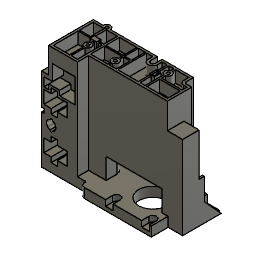
rightStepperBracket (Autodesk Fusion 360 design; units mm, degrees)
Autodesk Fusion 360 part; units mm, degrees
(part 1 of 3)
sketch "Sketch1" plane through (0, 0, 0) normal (0, 0, 1) x (1, 0, 0)
  line L0 (0, 0) -> (111.4, 0)
  line L1 (111.4, 0) -> (111.4, 93.5)
  line L2 (111.4, 93.5) -> (0, 93.5)
  line L3 (0, 93.5) -> (0, 0)
  line L4 (0, 71.5) -> (6, 71.5)
  line L5 (6, 71.5) -> (6, 93.5)
  line L6 (6, 93.5) -> (0, 93.5)
  line L7 (0, 93.5) -> (0, 71.5)
  line L8 (98.4, 93.5) -> (111.4, 93.5)
  line L9 (111.4, 93.5) -> (111.4, 71.5)
  line L10 (111.4, 71.5) -> (98.4, 71.5)
  line L11 (98.4, 71.5) -> (98.4, 93.5)
  line L12 (45.8, 8.3) -> (93.7, 8.3)
  line L13 (93.7, 8.3) -> (93.7, 26.1)
  line L14 (93.7, 26.1) -> (45.8, 26.1)
  line L15 (45.8, 26.1) -> (45.8, 8.3)
  line L16 (1.95, 58.65) -> (21.95, 58.65)
  line L17 (21.95, 58.65) -> (21.95, 47.65)
  line L18 (21.95, 47.65) -> (1.95, 47.65)
  line L19 (1.95, 47.65) -> (1.95, 58.65)
  line L20 (1.95, 22.7) -> (21.95, 22.7)
  line L21 (21.95, 22.7) -> (21.95, 11.7)
  line L22 (21.95, 11.7) -> (1.95, 11.7)
  line L23 (1.95, 11.7) -> (1.95, 22.7)
  point P0 (45.8, 17.2)
  point P1 (21.95, 17.2)
  dimension "d1" = 111.4
  dimension "d2" = 93.5
  dimension "d3" = 22
  dimension "d4" = 13
  dimension "d5" = 22
  dimension "d6" = 6
  dimension "d7" = 20
  dimension "d8" = 11
  dimension "d9" = 1.95
  dimension "d10" = 12.85
  dimension "d11" = 24.95
  dimension "d12" = 17.7
  dimension "d13" = 8.3
  dimension "d15" = 17.8
  dimension "d16" = 47.9
  constraint horizontal L0
  constraint vertical L1
  constraint horizontal L2
  constraint vertical L3
  constraint coincident L0.start L3.end
  constraint horizontal L4
  constraint vertical L5
  constraint horizontal L6
  constraint vertical L7
  constraint coincident L2 L5.end
  constraint coincident L3 L4.start
  constraint horizontal L8
  constraint vertical L9
  constraint horizontal L10
  constraint vertical L11
  constraint coincident L1 L9.end
  constraint coincident L2 L8.start
  constraint horizontal L12
  constraint vertical L13
  constraint horizontal L14
  constraint vertical L15
  constraint horizontal L16
  constraint vertical L17
  constraint horizontal L18
  constraint vertical L19
  constraint horizontal L20
  constraint vertical L21
  constraint horizontal L22
  constraint vertical L23
  constraint vertical L16.start L20.start
  constraint equal L16 L20
  constraint equal L17 L21
  constraint midpoint L15 P0
  constraint midpoint L21 P1
  constraint horizontal P0 P1
  measures "d1" distance of L0.start L0.end
  measures "d2" distance of L0.start L2.end
  measures "d3" distance of L8.start L10.end
  measures "d4" distance of L9.end L10.end
  measures "d5" distance of L4.end L5.end
  measures "d6" distance of L4.start L4.end
  measures "d7" distance of L16.start L16.end
  measures "d8" distance of L16.end L17.end
  measures "d9" distance of L3 L19
  measures "d10" distance of L4 L16
  measures "d11" distance of L18 L20
  measures "d12" distance of L1 L13
  measures "d13" distance of L0 L12
  measures "d15" distance of L12 L14
  measures "d16" distance of L13 L15
extrude "Extrude1" add sketch "Sketch1" along normal blind 42.8 contours L0 L1 L2 L3 L4 L5 L10 L11
sketch "Sketch2" plane through (0, 0, 42.8) normal (0, 0, 1) x (1, 0, 0)
  line L0 (21.95, 47.65) -> (1.95, 47.65)
  line L1 (1.95, 47.65) -> (1.95, 58.65)
  line L2 (1.95, 58.65) -> (21.95, 58.65)
  line L3 (21.95, 58.65) -> (21.95, 47.65)
  line L4 (45.8, 8.3) -> (45.8, 26.1)
  line L5 (45.8, 26.1) -> (93.7, 26.1)
  line L6 (93.7, 26.1) -> (93.7, 8.3)
  line L7 (93.7, 8.3) -> (45.8, 8.3)
  line L8 (21.95, 11.7) -> (1.95, 11.7)
  line L9 (1.95, 11.7) -> (1.95, 22.7)
  line L10 (1.95, 22.7) -> (21.95, 22.7)
  line L11 (21.95, 22.7) -> (21.95, 11.7)
  line L12 (0, 71.5) -> (0, 0)
  line L13 (0, 0) -> (111.4, 0)
  line L14 (111.4, 0) -> (111.4, 71.5)
  line L15 (111.4, 71.5) -> (98.4, 71.5)
  line L16 (98.4, 71.5) -> (98.4, 93.5)
  line L17 (98.4, 93.5) -> (6, 93.5)
  line L18 (6, 93.5) -> (6, 71.5)
  line L19 (6, 71.5) -> (0, 71.5)
  line L20 (30.75, 93.5) -> (111.4, 93.5)
  line L21 (111.4, 93.5) -> (111.4, 8.3)
  line L22 (111.4, 8.3) -> (30.75, 8.3)
  line L23 (30.75, 8.3) -> (30.75, 93.5)
  line L24 (38.2, 8.3) -> (99, 8.3)
  line L25 (99, 8.3) -> (99, 0)
  line L26 (99, 0) -> (38.2, 0)
  line L27 (38.2, 0) -> (38.2, 8.3)
  dimension "d19" = 30.75
  dimension "d23" = 12.4
  dimension "d24" = 60.8
  constraint horizontal L20
  constraint vertical L21
  constraint horizontal L22
  constraint vertical L23
  constraint coincident L14 L21.end
  constraint coincident L17 L20.start
  constraint collinear L7 L22
  constraint horizontal L24
  constraint vertical L25
  constraint horizontal L26
  constraint vertical L27
  constraint coincident L13 L25.end
  constraint coincident L22 L24.start
  measures "d19" distance of L12 L23
  measures "d23" distance of L14 L25
  measures "d24" distance of L25.end L26.end
extrude "Extrude2" cut sketch "Sketch2" against normal blind 9.5 contours L4 L5 L6 L14 L15 L16 L17 L20 L21 L22 L23 L24 | L13 L14 L22 L25
extrude "Extrude3" add sketch "Sketch2" along normal blind 5 contours L7 L13 L22 L24 L25 L26 L27
sketch "Sketch3" plane through (0, 0, 42.8) normal (0, 0, 1) x (1, 0, 0)
  line L0 (38.2, 0) -> (38.2, 8.3)
  line L1 (38.2, 8.3) -> (30.75, 8.3)
  line L2 (30.75, 8.3) -> (30.75, 93.5)
  line L3 (30.75, 93.5) -> (6, 93.5)
  line L4 (6, 93.5) -> (6, 71.5)
  line L5 (6, 71.5) -> (0, 71.5)
  line L6 (0, 71.5) -> (0, 0)
  line L7 (0, 0) -> (38.2, 0)
  line L8 (21.95, 47.65) -> (1.95, 47.65)
  line L9 (1.95, 47.65) -> (1.95, 58.65)
  line L10 (1.95, 58.65) -> (21.95, 58.65)
  line L11 (21.95, 58.65) -> (21.95, 47.65)
  line L12 (21.95, 11.7) -> (1.95, 11.7)
  line L13 (1.95, 11.7) -> (1.95, 22.7)
  line L14 (1.95, 22.7) -> (21.95, 22.7)
  line L15 (21.95, 22.7) -> (21.95, 11.7)
  line L16 (8.2, 58.65) -> (13.55, 58.65)
  line L17 (13.55, 58.65) -> (13.55, 62.9)
  line L18 (13.55, 62.9) -> (8.2, 62.9)
  line L19 (8.2, 62.9) -> (8.2, 58.65)
  line L20 (8.2, 47.65) -> (13.55, 47.65)
  line L21 (13.55, 47.65) -> (13.55, 43.4)
  line L22 (13.55, 43.4) -> (8.2, 43.4)
  line L23 (8.2, 43.4) -> (8.2, 47.65)
  line L24 (8.2, 22.7) -> (13.55, 22.7)
  line L25 (13.55, 22.7) -> (13.55, 26.95)
  line L26 (13.55, 26.95) -> (8.2, 26.95)
  line L27 (8.2, 26.95) -> (8.2, 22.7)
  line L28 (8.2, 11.7) -> (13.55, 11.7)
  line L29 (13.55, 11.7) -> (13.55, 7.45)
  line L30 (13.55, 7.45) -> (8.2, 7.45)
  line L31 (8.2, 7.45) -> (8.2, 11.7)
  circle A0 centre (8.25, 35.175) radius 4
  line L32 (21.95, 47.65) -> (21.95, 22.7) construction
  line L33 (9.3, 68.2) -> (2, 68.2)
  line L34 (2, 68.2) -> (2, 60.65)
  line L35 (2, 60.65) -> (6.2, 60.65)
  line L36 (6.2, 60.65) -> (6.2, 64.9)
  line L37 (6.2, 64.9) -> (15.55, 64.9)
  line L38 (28.75, 81.5) -> (9.3, 81.5)
  line L39 (9.3, 81.5) -> (9.3, 68.2)
  line L40 (28.75, 81.5) -> (28.75, 60.65)
  line L41 (28.75, 60.65) -> (15.55, 60.65)
  line L42 (15.55, 60.65) -> (15.55, 64.9)
  circle A1 centre (8.25, 31.175) radius 1
  circle A2 centre (8.25, 39.175) radius 1
  circle A3 centre (8.25, 35.175) radius 1.5
  line L43 (6.125, 39.175) -> (10.375, 39.175)
  line L44 (10.375, 39.175) -> (10.375, 31.175)
  line L45 (10.375, 31.175) -> (6.125, 31.175)
  line L46 (6.125, 31.175) -> (6.125, 39.175)
  point P0 (11.95, 7.2)
  point P1 (11.95, 11.45)
  point P2 (11.95, 26.7)
  point P3 (11.95, 22.45)
  point P4 (11.95, 62.9)
  point P5 (11.95, 58.65)
  point P6 (11.95, 43.4)
  point P7 (11.95, 47.65)
  point P8 (21.95, 35.175)
  point P9 (8.25, 39.175)
  point P10 (8.25, 31.175)
  dimension "d27" = 5.35
  dimension "d28" = 19.5
  dimension "d29" = 8.2
  dimension "d30" = 8
  dimension "d31" = 8.25
  dimension "d32" = 12
  dimension "d33" = 2
  dimension "d34" = 2
  dimension "d35" = 2
  dimension "d36" = 2
  dimension "d37" = 2
  dimension "d38" = 2
  dimension "d39" = 2
  dimension "d40" = 3.3
  dimension "d41" = 3.3
  dimension "d47" = 2
  dimension "d48" = 2
  dimension "d49" = 3
  dimension "d50" = 4.25
  constraint horizontal L16
  constraint vertical L17
  constraint horizontal L18
  constraint vertical L19
  constraint coincident L10 L16.start
  constraint horizontal L20
  constraint vertical L21
  constraint horizontal L22
  constraint vertical L23
  constraint coincident L8 L20.start
  constraint horizontal L24
  constraint vertical L25
  constraint horizontal L26
  constraint vertical L27
  constraint coincident L14 L24.start
  constraint horizontal L28
  constraint vertical L29
  constraint horizontal L30
  constraint vertical L31
  constraint coincident L12 L28.start
  constraint vertical P0 P1
  constraint vertical P2 P3
  constraint vertical P4 P5
  constraint vertical P6 P7
  constraint equal L18 L22
  constraint equal L17 L21
  constraint equal L21 L25
  constraint equal L25 L29
  constraint equal L24 L30
  constraint equal L18 L26
  constraint vertical L24.start L28.start
  constraint vertical L22.end L26.end
  constraint vertical L16.start L20.start
  constraint coincident L8.start L11.end
  constraint coincident L14.end L15.start
  constraint midpoint L32 P8
  constraint horizontal A0.centre P8
  constraint horizontal L33
  constraint perpendicular L33 L34
  constraint perpendicular L34 L35
  constraint perpendicular L33 L36
  constraint perpendicular L36 L37
  constraint perpendicular L33 L39
  constraint perpendicular L37 L40
  constraint perpendicular L17 L41
  constraint perpendicular L37 L42
  constraint coincident L38.start L40.start
  constraint coincident A0 P10
  constraint coincident A0 P9
  constraint vertical A0.centre P9
  constraint vertical A0.centre P10
  constraint concentric A0 A3
  constraint horizontal L43
  constraint vertical L44
  constraint horizontal L45
  constraint vertical L46
  constraint midpoint L43 P9
  constraint coincident P9 A2.centre
  constraint midpoint L45 P10
  constraint coincident P10 A1.centre
  measures "d27" distance of L17.end L18.end
  measures "d28" distance of L18 L22
  measures "d29" distance of L6 L27
  measures "d30" diameter of A0
  measures "d31" distance of L6 A0.centre
  measures "d32" distance of L3 L38
  measures "d33" distance of L6 L34
  measures "d34" distance of L10 L35
  measures "d35" distance of L19 L36
  measures "d36" distance of L18 L37
  measures "d37" distance of L17 L42
  measures "d38" distance of L10 L41
  measures "d39" distance of L2 L40
  measures "d40" distance of L5 L33
  measures "d41" distance of L4 L39
  measures "d47" diameter of A1
  measures "d48" diameter of A2
  measures "d49" diameter of A3
  measures "d50" distance of L44 L46
extrude "Extrude4" cut sketch "Sketch3" against normal blind 29 contours L8 L20 L21 L22 L23 | L10 L16 L17 L18 L19 | L12 L28 L29 L30 L31 | L14 L24 L25 L26 L27
extrude "Extrude5" cut sketch "Sketch3" against normal blind 9.6 contours L33 L34 L35 L36 L37 L38 L39 L40 L41 L42
extrude "Extrude6" cut sketch "Sketch3" against normal blind 25 contours A0 A1 A2 L44 L46 | A0 A2 | A0 A2 L43 | A0 A1 L45 | A0 A1 | A0 A2 L43 | A2 L43 | A0 A1 L45 | A1 L45 | A3
extrude "Extrude7" cut sketch "Sketch3" against normal up to surface (42.8 mm away) contours A3
extrude "Extrude8" cut sketch "Sketch3" against normal blind 15.15 contours A0 L44 | A0 L46
sketch "Sketch4" plane through (0, 0, 0) normal (0, 0, -1) x (-1, 0, 0)
  circle A0 centre (-8.25, 35.175) radius 1.5
  line L0 (-1.95, 47.65) -> (-21.95, 47.65)
  line L1 (-21.95, 47.65) -> (-21.95, 58.65)
  line L2 (-21.95, 58.65) -> (-1.95, 58.65)
  line L3 (-1.95, 58.65) -> (-1.95, 47.65)
  line L4 (-45.8, 26.1) -> (-45.8, 8.3)
  line L5 (-45.8, 8.3) -> (-93.7, 8.3)
  line L6 (-93.7, 8.3) -> (-93.7, 26.1)
  line L7 (-93.7, 26.1) -> (-45.8, 26.1)
  line L8 (-1.95, 11.7) -> (-21.95, 11.7)
  line L9 (-21.95, 11.7) -> (-21.95, 22.7)
  line L10 (-21.95, 22.7) -> (-1.95, 22.7)
  line L11 (-1.95, 22.7) -> (-1.95, 11.7)
  line L12 (0, 0) -> (0, 71.5)
  line L13 (0, 71.5) -> (-6, 71.5)
  line L14 (-6, 71.5) -> (-6, 93.5)
  line L15 (-6, 93.5) -> (-98.4, 93.5)
  line L16 (-98.4, 93.5) -> (-98.4, 71.5)
  line L17 (-98.4, 71.5) -> (-111.4, 71.5)
  line L18 (-111.4, 71.5) -> (-111.4, 0)
  line L19 (-111.4, 0) -> (0, 0)
  line L20 (-97.3, 1.8) -> (-40.3, 1.8)
  line L21 (-40.3, 1.8) -> (-40.3, 32.85)
  line L22 (-97.3, 32.85) -> (-97.3, 1.8)
  circle A1 centre (-68.565, 5.235) radius 1.2
  circle A2 centre (-57.165, 5.235) radius 1.2
  line L23 (-97.3, 32.85) -> (-40.3, 32.85)
  circle A3 centre (-68.565, 29.235) radius 1.2
  circle A4 centre (-57.165, 29.235) radius 1.2
  circle A5 centre (-68.565, 29.235) radius 3.3
  circle A6 centre (-57.165, 29.235) radius 3.3
  circle A7 centre (-68.565, 5.235) radius 3.3
  circle A8 centre (-57.165, 5.235) radius 3.3
  dimension "d57" = 14.1
  dimension "d58" = 57
  dimension "d59" = 1.8
  dimension "d60" = 11.4
  dimension "d61" = 28.735
  dimension "d63" = 3.065
  dimension "d64" = 2.4
  dimension "d65" = 6.75
  dimension "d67" = 6.6
  dimension "d68" = 24
  constraint horizontal L20
  constraint vertical L21
  constraint vertical L22
  constraint equal A1 A2
  constraint horizontal A1.centre A2.centre
  constraint perpendicular L22 L23
  constraint vertical A1.centre A3.centre
  constraint vertical A2.centre A4.centre
  constraint horizontal A3.centre A4.centre
  constraint equal A3 A4
  constraint equal A1 A3
  constraint concentric A3 A5
  constraint concentric A4 A6
  constraint equal A5 A6
  constraint concentric A1 A7
  constraint concentric A2 A8
  constraint equal A6 A8
  constraint equal A7 A8
  measures "d57" distance of L18 L22
  measures "d58" distance of L21 L22
  measures "d59" distance of L19 L20
  measures "d60" distance of A1.centre A2.centre
  measures "d61" distance of L22 A1.centre
  measures "d63" distance of L5 A1.centre
  measures "d64" diameter of A1
  measures "d65" distance of L7 L23
  measures "d67" diameter of A5
  measures "d68" distance of A1.centre A3.centre
extrude "Extrude9" cut sketch "Sketch4" against normal blind 2 contours L7 A6 | L5 A8 | L7 A5 | L5 A7 | L20 L21 L22 L23 | A1 | A2 | A3 | A4 picked at (-57.1351, 26.7461) picked at (-57.1949, 7.6772) picked at (-68.5949, 26.7461) picked at (-68.5949, 7.6772)
extrude "Extrude10" cut sketch "Sketch4" against normal blind 9 from surface at -2 contours A1 | A2 | A3 | A4
sketch "Sketch6" plane through (0, 0, 0) normal (0, 0, -1) x (-1, 0, 0)
  line L0 (-40.3, 32.85) -> (-40.3, 1.8)
  line L1 (-40.3, 1.8) -> (-97.3, 1.8)
  line L2 (-97.3, 1.8) -> (-97.3, 32.85)
  line L3 (-97.3, 32.85) -> (-40.3, 32.85)
  circle A0 centre (-8.25, 35.175) radius 1.5
  line L4 (-1.95, 47.65) -> (-21.95, 47.65)
  line L5 (-21.95, 47.65) -> (-21.95, 58.65)
  line L6 (-21.95, 58.65) -> (-1.95, 58.65)
  line L7 (-1.95, 58.65) -> (-1.95, 47.65)
  line L8 (-1.95, 11.7) -> (-21.95, 11.7)
  line L9 (-21.95, 11.7) -> (-21.95, 22.7)
  line L10 (-21.95, 22.7) -> (-1.95, 22.7)
  line L11 (-1.95, 22.7) -> (-1.95, 11.7)
  line L12 (0, 0) -> (0, 71.5)
  line L13 (0, 71.5) -> (-6, 71.5)
  line L14 (-6, 71.5) -> (-6, 93.5)
  line L15 (-6, 93.5) -> (-98.4, 93.5)
  line L16 (-98.4, 93.5) -> (-98.4, 71.5)
  line L17 (-98.4, 71.5) -> (-111.4, 71.5)
  line L18 (-111.4, 71.5) -> (-111.4, 0)
  line L19 (-111.4, 0) -> (0, 0)
  line L20 (-98.4, 71.5) -> (-98.4, 26.1)
  line L21 (-98.4, 26.1) -> (-93.7, 26.1)
  line L22 (-93.7, 26.1) -> (-93.7, 8.3)
  line L23 (-93.7, 8.3) -> (-99.3, 8.3)
  line L24 (-99.3, 8.3) -> (-99.3, 1.6)
  line L25 (-99.3, 1.6) -> (-109.65, 1.6)
  line L26 (-109.65, 1.6) -> (-109.65, 34.9)
  line L27 (-109.65, 34.9) -> (-111.4, 34.9)
  point P0 (-93.7, 8.3)
  point P1 (-93.7, 26.1)
  dimension "d80" = 34.9
  dimension "d81" = 1.75
  dimension "d82" = 1.6
  dimension "d83" = 2
  constraint coincident L16.end L17.start
  constraint perpendicular L17 L20
  constraint coincident P1 L21.end
  constraint perpendicular L2 L21
  constraint coincident P0 L22.end
  constraint perpendicular L2 L23
  constraint perpendicular L23 L24
  constraint perpendicular L2 L25
  constraint perpendicular L25 L26
  constraint coincident L18 L27.end
  constraint perpendicular L18 L27
  measures "d80" distance of L18.end L27.end
  measures "d81" distance of L18 L26
  measures "d82" distance of L19 L25
  measures "d83" distance of L2 L24
extrude "Extrude11" cut sketch "Sketch6" against normal blind 19.1 contours L2 L21 L22 L23 | L2 L17 L18 L20 L21 L23 L24 L25 L26 L27
sketch "Sketch5" plane through (0, 8.3, 0) normal (0, 1, 0) x (-1, 0, 0)
  line L0 (-97.3, 2) -> (-45.8, 2)
  line L1 (-45.8, 2) -> (-45.8, 33.3)
  line L2 (-45.8, 33.3) -> (-30.75, 33.3)
  line L3 (-30.75, 33.3) -> (-30.75, 42.8)
  line L4 (-30.75, 42.8) -> (-38.2, 42.8)
  line L5 (-38.2, 42.8) -> (-38.2, 47.8)
  line L6 (-38.2, 47.8) -> (-99, 47.8)
  line L7 (-99, 47.8) -> (-99, 33.3)
  line L8 (-99, 33.3) -> (-93.7, 33.3)
  line L9 (-93.7, 33.3) -> (-93.7, 19.1)
  circle A0 centre (-78.55, 26.05) radius 12
  circle A1 centre (-63.05, 41.55) radius 1.75
  circle A2 centre (-94.05, 41.55) radius 1.75
  circle A3 centre (-94.05, 10.55) radius 1.75
  circle A4 centre (-63.05, 10.55) radius 1.75
  line L10 (-63.05, 10.55) -> (-63.05, 41.55) construction
  line L11 (-63.05, 41.55) -> (-94.05, 41.55) construction
  line L12 (-111.4, 0) -> (-111.4, 33.3) construction
  line L13 (-93.7, 19.1) -> (-99.3, 19.1)
  line L14 (-99.3, 19.1) -> (-99.3, 0)
  line L15 (-99.3, 0) -> (-97.3, 0)
  line L16 (-97.3, 0) -> (-97.3, 2)
  circle A5 centre (-63.05, 41.55) radius 3.25
  circle A6 centre (-94.05, 41.55) radius 3.25
  circle A7 centre (-94.05, 10.55) radius 3.25
  circle A8 centre (-63.05, 10.55) radius 3.25
  line L17 (-59.8, 10.55) -> (-59.8, 2)
  line L18 (-66.3, 10.55) -> (-66.3, 2)
  line L19 (-59.8, 41.55) -> (-59.8, 47.8)
  line L20 (-66.3, 41.55) -> (-66.3, 47.8)
  line L21 (-90.8, 41.55) -> (-90.8, 47.8)
  line L22 (-97.3, 41.55) -> (-97.3, 47.8)
  line L23 (-97.3, 10.55) -> (-97.3, 0)
  line L24 (-90.8, 10.55) -> (-90.8, 2)
  point P0 (-63.05, 26.05)
  point P1 (-78.55, 41.55)
  dimension "d75" = 24
  dimension "d76" = 3.5
  dimension "d86" = 6.5
  dimension "d87" = 6.25
  dimension "d88" = 31
  constraint equal A3 A4
  constraint equal A1 A4
  constraint equal A1 A2
  constraint horizontal A3.centre A4.centre
  constraint vertical A2.centre A3.centre
  constraint horizontal A1.centre A2.centre
  constraint vertical A1.centre A4.centre
  constraint coincident A4.centre L10.start
  constraint coincident A1.centre L10.end
  constraint coincident A2.centre L11.end
  constraint midpoint L10 P0
  constraint horizontal A0.centre P0
  constraint midpoint L11 P1
  constraint vertical A0.centre P1
  constraint equal L10 L11
  constraint concentric A3 A7
  constraint equal A7 A8
  constraint equal A6 A7
  constraint equal A5 A6
  constraint coincident A8 L17.start
  constraint coincident L0 L17.end
  constraint tangent A8 L17
  constraint perpendicular L0 L17
  constraint coincident A8 L18.start
  constraint coincident L0 L18.end
  constraint tangent A8 L18
  constraint perpendicular L0 L18
  constraint coincident A5 L19.start
  constraint coincident L6 L19.end
  constraint tangent A5 L19
  constraint perpendicular L6 L19
  constraint coincident A5 L20.start
  constraint coincident L11 L20.start
  constraint coincident L6 L20.end
  constraint tangent A5 L20
  constraint coincident L11 L21.start
  constraint coincident A6 L21.start
  constraint coincident L6 L21.end
  constraint tangent A6 L21
  constraint coincident A6 L22.start
  constraint coincident L6 L22.end
  constraint tangent A6 L22
  constraint perpendicular L6 L22
  constraint coincident A7 L23.start
  constraint coincident L15.end L16.start
  constraint perpendicular L0 L23
  constraint coincident A7 L24.start
  constraint coincident L0 L24.end
  constraint tangent A7 L24
  constraint perpendicular L0 L24
  measures "d75" diameter of A0
  measures "d76" diameter of A4
  measures "d86" diameter of A5
  measures "d87" distance of L19.start L19.end
  measures "d88" distance of A1.centre A2.centre
extrude "Extrude12" cut sketch "Sketch5" against normal up to surface (8.3 mm away) contours A0 | A1 | A2 | A3 | A4
extrude "Extrude13" cut sketch "Sketch5" against normal blind 4.9 contours L0 A7 L23 L24 | A7 | L0 A8 L17 L18 | A8 | L6 A6 L21 L22 | A6 | L6 A5 L19 L20 | A5
sketch "Sketch7" plane through (0, 58.65, 0) normal (0, -1, 0) x (1, 0, 0)
  line L0 (8.2, 13.8) -> (8.2, 42.8)
  line L1 (8.2, 42.8) -> (1.95, 42.8)
  line L2 (1.95, 42.8) -> (1.95, 0)
  line L3 (1.95, 0) -> (21.95, 0)
  line L4 (21.95, 0) -> (21.95, 42.8)
  line L5 (21.95, 42.8) -> (13.55, 42.8)
  line L6 (13.55, 42.8) -> (13.55, 13.8)
  line L7 (13.55, 13.8) -> (8.2, 13.8)
  circle A0 centre (10.875, 8.975) radius 2.525
  line L8 (13.4, 8.975) -> (13.4, 0)
  line L9 (8.35, 8.975) -> (8.35, 0)
  circle A1 centre (10.875, 10.3) radius 3.5
  line L10 (13.55, 13.8) -> (13.55, 12.5571)
  line L11 (8.2, 13.8) -> (8.2, 12.5571)
  line L12 (11.625, 11.5) -> (10.125, 11.5)
  line L13 (10.125, 11.5) -> (10.125, 5)
  line L14 (10.125, 5) -> (11.625, 5)
  line L15 (11.625, 5) -> (11.625, 11.5)
  line L16 (8.35, 0) -> (13.4, 0) construction
  line L17 (13.4, 0) -> (8.35, 0) construction
  point P0 (10.875, 5)
  point P1 (10.875, 0)
  point P2 (10.875, 13.8)
  dimension "d93" = 5.05
  dimension "d94" = 8.975
  dimension "d95" = 7
  dimension "d96" = 1.5
  dimension "d97" = 6.5
  constraint coincident A0 L8.start
  constraint coincident L3 L8.end
  constraint tangent A0 L8
  constraint perpendicular L3 L8
  constraint coincident A0 L9.start
  constraint coincident L3 L9.end
  constraint tangent A0 L9
  constraint perpendicular L3 L9
  constraint tangent L7 A1
  constraint coincident L6.end L7.start
  constraint coincident A1 L10.end
  constraint perpendicular L7 L10
  constraint coincident L0.start L7.end
  constraint coincident A1 L11.end
  constraint perpendicular L7 L11
  constraint horizontal L12
  constraint vertical L13
  constraint horizontal L14
  constraint vertical L15
  constraint tangent A0 L12
  constraint midpoint L14 P0
  constraint vertical A0.centre P0
  constraint midpoint L17 P1
  constraint midpoint L7 P2
  constraint vertical P1 P2
  constraint vertical A1.centre P1
  measures "d93" diameter of A0
  measures "d94" distance of L8.start L8.end
  measures "d95" diameter of A1
  measures "d96" distance of L13.end L14.end
  measures "d97" distance of L12.end L13.end
extrude "Extrude14" cut sketch "Sketch7" against normal blind 4 contours L7 A1 L11 | L7 A1 L10 | L3 A0 L8 L9 A1 L13 L14 L15 | A0 L9 A1 | A0 A1 L13 | A0 A1 L13 | A0 L8 A1 | A0 A1 L13 L15 | A0 A1 L13 L15 | A0 L13 L14 L15 | A0 A1 L15 | A0 A1 L15
extrude "Extrude15" cut 2 faces at (13.1796, 62.65, 13.3159) (8.5704, 62.65, 13.3159) along direction (0, -1, 0) up to surface end surface through (13.55, 62.9, 42.8) normal (0, -1, 0) offset 0
extrude "Extrude16" add sketch "Sketch7" along normal blind 0.95 from surface at -4 contours A0 A1 L13 L15 | A0 A1 L13 L15 | A0 L13 L14 L15
chamfer "Chamfer1" distance 0.95 angle 45 1 edges at (10.875, 61.7, 5)
sketch "Sketch8" plane through (0, 22.7, 0) normal (0, -1, 0) x (1, 0, 0)
  line L0 (8.2, 13.8) -> (8.2, 42.8)
  line L1 (8.2, 42.8) -> (1.95, 42.8)
  line L2 (1.95, 42.8) -> (1.95, 0)
  line L3 (1.95, 0) -> (21.95, 0)
  line L4 (21.95, 0) -> (21.95, 42.8)
  line L5 (21.95, 42.8) -> (13.55, 42.8)
  line L6 (13.55, 42.8) -> (13.55, 13.8)
  line L7 (13.55, 13.8) -> (8.2, 13.8)
  line L8 (11.625, 5) -> (11.625, 11.5)
  line L9 (11.625, 11.5) -> (10.125, 11.5)
  line L10 (8.2, 13.8) -> (8.2, 12.5571)
  line L11 (10.125, 11.5) -> (10.125, 5)
  line L12 (13.55, 13.8) -> (13.55, 12.5571)
  circle A0 centre (10.875, 8.975) radius 2.525
  line L13 (13.55, 13.8) -> (8.2, 13.8)
  line L14 (13.4, 8.975) -> (13.4, 0)
  circle A1 centre (10.875, 10.3) radius 3.5
  line L15 (8.35, 8.975) -> (8.35, 0)
  line L16 (10.125, 5) -> (11.625, 5)
  line L17 (8.35, 0) -> (13.4, 0) construction
  point P0 (10.875, 5)
  point P1 (13.55, 13.8)
  point P2 (10.875, 0)
  point P3 (10.875, 13.8)
  dimension "d106" = 5.05
  dimension "d107" = 8.975
  dimension "d108" = 7
  dimension "d109" = 1.5
  dimension "d110" = 6.5
  constraint coincident L14.start A0
  constraint tangent A0 L14
  constraint coincident L15.start A0
  constraint tangent A0 L15
  constraint tangent L13 A1
  constraint coincident P1 L6.end
  constraint coincident L12.end A1
  constraint perpendicular L12 L13
  constraint coincident L0.start L7.end
  constraint coincident L10.end A1
  constraint perpendicular L10 L13
  constraint horizontal L9
  constraint vertical L11
  constraint horizontal L16
  constraint vertical L8
  constraint tangent L9 A0
  constraint midpoint P0 L16
  constraint vertical A0.centre P0
  constraint coincident L3 L14.end
  constraint coincident L3 L15.end
  constraint vertical A0.centre A1.centre
  constraint coincident L0 L7.end
  constraint collinear L0 L10
  constraint perpendicular L3 L14
  constraint perpendicular L3 L15
  constraint midpoint L17 P2
  constraint midpoint L7 P3
  constraint vertical P2 P3
  measures "d106" diameter of A0
  measures "d107" distance of L14.start L14.end
  measures "d108" diameter of A1
  measures "d109" distance of L11.end L8.start
  measures "d110" distance of L11.end L9.end
extrude "Extrude17" cut sketch "Sketch8" against normal blind 4 contours L7 L10 L13 A1 | L7 L12 L13 A1 | A0 A1 L15 | L3 L8 L11 A0 L14 A1 L15 L16 | L11 A0 A1 | L11 A0 A1 | A0 L14 A1 | L8 L11 A0 L16 | L8 L11 A0 A1 | L8 L11 A0 A1 | L8 A0 A1 | L8 A0 A1
extrude "Extrude18" cut 2 faces at (13.1796, 26.7, 13.3159) (8.5704, 26.7, 13.3159) along direction (0, -1, 0) up to surface end surface through (13.55, 26.95, 42.8) normal (0, -1, 0) offset 0
extrude "Extrude19" add sketch "Sketch8" along normal blind 0.95 from surface at -4 contours L8 L11 A0 L16 | L8 L11 A0 A1 | L8 L11 A0 A1
chamfer "Chamfer2" distance 0.95 angle 45 1 edges at (10.875, 25.75, 5)
sketch "Sketch9" plane through (0, 11.7, 0) normal (0, 1, 0) x (-1, 0, 0)
  line L0 (-8.2, 42.8) -> (-8.2, 13.8)
  line L1 (-8.2, 13.8) -> (-13.55, 13.8)
  line L2 (-13.55, 13.8) -> (-13.55, 42.8)
  line L3 (-13.55, 42.8) -> (-21.95, 42.8)
  line L4 (-21.95, 42.8) -> (-21.95, 0)
  line L5 (-21.95, 0) -> (-1.95, 0)
  line L6 (-1.95, 0) -> (-1.95, 42.8)
  line L7 (-1.95, 42.8) -> (-8.2, 42.8)
  line L8 (-13.55, 13.8) -> (-13.55, 12.5571)
  line L9 (-13.4, 8.975) -> (-13.4, 0)
  line L10 (-8.2, 13.8) -> (-13.55, 13.8)
  circle A0 centre (-10.875, 8.975) radius 2.525
  line L11 (-10.125, 5) -> (-10.125, 11.5)
  line L12 (-8.35, 8.975) -> (-8.35, 0)
  line L13 (-11.625, 5) -> (-10.125, 5)
  line L14 (-10.125, 11.5) -> (-11.625, 11.5)
  line L15 (-8.2, 13.8) -> (-8.2, 12.5571)
  line L16 (-11.625, 11.5) -> (-11.625, 5)
  line L17 (-13.4, 0) -> (-8.35, 0) construction
  circle A1 centre (-10.875, 10.3) radius 3.5
  point P0 (-10.875, 13.8)
  point P1 (-10.875, 0)
  point P2 (-8.2, 13.8)
  point P3 (-10.875, 5)
  point P4 (-10.875, 13.8)
  dimension "d119" = 5.05
  dimension "d120" = 8.975
  dimension "d121" = 7
  dimension "d122" = 1.5
  dimension "d123" = 6.5
  constraint coincident L12.start A0
  constraint tangent A0 L12
  constraint coincident L9.start A0
  constraint tangent L9 A0
  constraint tangent L10 A1
  constraint coincident P2 L0.end
  constraint coincident L15.end A1
  constraint perpendicular L10 L15
  constraint coincident L1.end L2.start
  constraint coincident L8.end A1
  constraint perpendicular L8 L10
  constraint horizontal L14
  constraint vertical L16
  constraint horizontal L13
  constraint vertical L11
  constraint tangent A0 L14
  constraint midpoint P3 L13
  constraint vertical P3 A0.centre
  constraint vertical A1.centre A0.centre
  constraint midpoint P1 L17
  constraint vertical P4 P1
  constraint perpendicular L12 L17
  constraint perpendicular L9 L17
  constraint collinear L5 L17
  constraint midpoint L1 P4
  constraint vertical P1 P4
  constraint coincident L0.end L1.start
  measures "d119" diameter of A0
  measures "d120" distance of L12.start L12.end
  measures "d121" diameter of A1
  measures "d122" distance of L13.start L11.start
  measures "d123" distance of L14.end L13.start
extrude "Extrude20" cut sketch "Sketch9" against normal blind 4 contours L1 L10 L15 A1 | L1 L8 L10 A1 | L5 L9 A0 L11 L12 L13 L16 A1 | L9 A0 A1 | A0 L12 A1 | A0 L16 A1 | A0 L16 A1 | A0 L11 A1 | A0 L11 A1 | A0 L11 L16 A1 | A0 L11 L16 A1 | A0 L11 L13 L16
extrude "Extrude21" cut 2 faces at (8.5704, 7.7, 13.3159) (13.1796, 7.7, 13.3159) along direction (0, 1, 0) up to surface end surface through (13.55, 7.45, 42.8) normal (0, 1, 0) offset 0
extrude "Extrude22" add sketch "Sketch9" along normal blind 0.95 from surface at -4 contours A0 L11 L16 A1 | A0 L11 L16 A1 | A0 L11 L13 L16
chamfer "Chamfer3" distance 0.95 angle 45 1 edges at (10.875, 8.65, 5)
sketch "Sketch10" plane through (0, 47.65, 0) normal (0, 1, 0) x (-1, 0, 0)
  line L0 (-8.2, 42.8) -> (-8.2, 13.8)
  line L1 (-8.2, 13.8) -> (-13.55, 13.8)
  line L2 (-13.55, 13.8) -> (-13.55, 42.8)
  line L3 (-13.55, 42.8) -> (-21.95, 42.8)
  line L4 (-21.95, 42.8) -> (-21.95, 0)
  line L5 (-21.95, 0) -> (-1.95, 0)
  line L6 (-1.95, 0) -> (-1.95, 42.8)
  line L7 (-1.95, 42.8) -> (-8.2, 42.8)
  line L8 (-10.125, 11.5) -> (-11.625, 11.5)
  line L9 (-11.625, 11.5) -> (-11.625, 5)
  line L10 (-13.4, 0) -> (-8.35, 0) construction
  line L11 (-8.35, 8.975) -> (-8.35, 0)
  circle A0 centre (-10.875, 8.975) radius 2.525
  line L12 (-13.4, 8.975) -> (-13.4, 0)
  line L13 (-10.125, 5) -> (-10.125, 11.5)
  line L14 (-8.2, 13.8) -> (-13.55, 13.8)
  line L15 (-11.625, 5) -> (-10.125, 5)
  line L16 (-13.55, 13.8) -> (-13.55, 12.5571)
  circle A1 centre (-10.875, 10.3) radius 3.5
  line L17 (-8.2, 13.8) -> (-8.2, 12.5571)
  point P0 (-8.2, 13.8)
  point P1 (-10.875, 0)
  point P2 (-10.875, 5)
  point P3 (-10.875, 13.8)
  point P4 (-10.875, 13.8)
  dimension "d132" = 5.05
  dimension "d133" = 8.975
  dimension "d134" = 7
  dimension "d135" = 1.5
  dimension "d136" = 6.5
  constraint coincident L11.start A0
  constraint tangent L11 A0
  constraint coincident L12.start A0
  constraint tangent A0 L12
  constraint tangent L14 A1
  constraint coincident P0 L0.end
  constraint coincident L17.end A1
  constraint perpendicular L14 L17
  constraint coincident L1.end L2.start
  constraint coincident L16.end A1
  constraint perpendicular L14 L16
  constraint horizontal L8
  constraint vertical L9
  constraint horizontal L15
  constraint vertical L13
  constraint tangent L8 A0
  constraint midpoint P2 L15
  constraint vertical A0.centre P2
  constraint vertical A0.centre A1.centre
  constraint midpoint P1 L10
  constraint perpendicular L10 L11
  constraint perpendicular L10 L12
  constraint vertical P1 P4
  constraint collinear L5 L10
  constraint midpoint L1 P4
  measures "d132" diameter of A0
  measures "d133" distance of L11.start L10.end
  measures "d134" diameter of A1
  measures "d135" distance of L13.start L9.end
  measures "d136" distance of L9.end L8.end
extrude "Extrude23" cut sketch "Sketch10" against normal blind 4 contours L1 L14 A1 L17 | L1 L14 L16 A1 | L5 L9 L11 A0 L12 L13 L15 A1 | A0 L12 A1 | L11 A0 A1 | L9 A0 A1 | L9 A0 A1 | A0 L13 A1 | A0 L13 A1 | L9 A0 L13 A1 | L9 A0 L13 L15 | L9 A0 L13 A1
extrude "Extrude24" cut 2 faces at (8.5704, 43.65, 13.3159) (13.1796, 43.65, 13.3159) along direction (0, 1, 0) up to surface end surface through (13.55, 43.4, 42.8) normal (0, 1, 0) offset 0
extrude "Extrude25" add sketch "Sketch10" along normal blind 0.95 from surface at -4 contours L9 A0 L13 A1 | L9 A0 L13 L15 | L9 A0 L13 A1
chamfer "Chamfer4" distance 0.95 angle 45 1 edges at (10.875, 44.6, 5)
sketch "Sketch11" plane through (0, 0, 0) normal (0, 0, -1) x (-1, 0, 0)
  circle A0 centre (-8.25, 35.175) radius 1.5
  line L0 (-8.35, 47.65) -> (-8.35, 43.65)
  line L1 (-8.35, 43.65) -> (-13.4, 43.65)
  line L2 (-13.4, 43.65) -> (-13.4, 47.65)
  line L3 (-13.4, 47.65) -> (-21.95, 47.65)
  line L4 (-21.95, 47.65) -> (-21.95, 58.65)
  line L5 (-21.95, 58.65) -> (-13.4, 58.65)
  line L6 (-13.4, 58.65) -> (-13.4, 62.65)
  line L7 (-13.4, 62.65) -> (-8.35, 62.65)
  line L8 (-8.35, 62.65) -> (-8.35, 58.65)
  line L9 (-8.35, 58.65) -> (-1.95, 58.65)
  line L10 (-1.95, 58.65) -> (-1.95, 47.65)
  line L11 (-1.95, 47.65) -> (-8.35, 47.65)
  line L12 (-97.3, 8.3) -> (-99.3, 8.3)
  line L13 (-99.3, 8.3) -> (-99.3, 1.6)
  line L14 (-99.3, 1.6) -> (-109.65, 1.6)
  line L15 (-109.65, 1.6) -> (-109.65, 34.9)
  line L16 (-109.65, 34.9) -> (-111.4, 34.9)
  line L17 (-111.4, 34.9) -> (-111.4, 0)
  line L18 (-111.4, 0) -> (0, 0)
  line L19 (0, 0) -> (0, 71.5)
  line L20 (0, 71.5) -> (-6, 71.5)
  line L21 (-6, 71.5) -> (-6, 93.5)
  line L22 (-6, 93.5) -> (-98.4, 93.5)
  line L23 (-98.4, 93.5) -> (-98.4, 26.1)
  line L24 (-98.4, 26.1) -> (-97.3, 26.1)
  line L25 (-97.3, 26.1) -> (-97.3, 32.85)
  line L26 (-97.3, 32.85) -> (-40.3, 32.85)
  line L27 (-40.3, 32.85) -> (-40.3, 1.8)
  line L28 (-40.3, 1.8) -> (-97.3, 1.8)
  line L29 (-97.3, 1.8) -> (-97.3, 8.3)
  line L30 (-13.4, 7.7) -> (-13.4, 11.7)
  line L31 (-13.4, 11.7) -> (-21.95, 11.7)
  line L32 (-21.95, 11.7) -> (-21.95, 22.7)
  line L33 (-21.95, 22.7) -> (-13.4, 22.7)
  line L34 (-13.4, 22.7) -> (-13.4, 26.7)
  line L35 (-13.4, 26.7) -> (-8.35, 26.7)
  line L36 (-8.35, 26.7) -> (-8.35, 22.7)
  line L37 (-8.35, 22.7) -> (-1.95, 22.7)
  line L38 (-1.95, 22.7) -> (-1.95, 11.7)
  line L39 (-1.95, 11.7) -> (-8.35, 11.7)
  line L40 (-8.35, 11.7) -> (-8.35, 7.7)
  line L41 (-8.35, 7.7) -> (-13.4, 7.7)
  line L42 (-98.4, 93.5) -> (-30.5, 93.5)
  line L43 (-30.5, 93.5) -> (-30.5, 34.2)
  line L44 (-30.5, 34.2) -> (-98.4, 34.2)
  line L45 (-98.4, 34.2) -> (-98.4, 93.5)
  line L46 (-21.95, 58.65) -> (-30.5, 58.65)
  line L47 (-21.95, 47.65) -> (-30.5, 47.65)
  dimension "d145" = 1.35
  dimension "d146" = 30.5
  constraint horizontal L42
  constraint vertical L43
  constraint horizontal L44
  constraint vertical L45
  constraint coincident L22.end L23.start
  constraint coincident L4.end L5.start
  constraint coincident L43 L46.end
  constraint perpendicular L43 L46
  constraint coincident L3.end L4.start
  constraint coincident L43 L47.end
  constraint perpendicular L43 L47
  measures "d145" distance of L26 L44
  measures "d146" distance of L19 L43
extrude "Extrude26" cut sketch "Sketch11" against normal blind 4.5 contours L4 L43 L46 L47 | L22 L23 L42 L43 L44 L45
sketch "Sketch12" plane through (0, 0, 0) normal (0, 0, -1) x (-1, 0, 0)
  line L0 (-30.5, 34.2) -> (-98.4, 34.2)
  line L1 (-98.4, 34.2) -> (-98.4, 26.1)
  line L2 (-98.4, 26.1) -> (-97.3, 26.1)
  line L3 (-97.3, 26.1) -> (-97.3, 32.85)
  line L4 (-97.3, 32.85) -> (-40.3, 32.85)
  line L5 (-40.3, 32.85) -> (-40.3, 1.8)
  line L6 (-40.3, 1.8) -> (-97.3, 1.8)
  line L7 (-97.3, 1.8) -> (-97.3, 8.3)
  line L8 (-97.3, 8.3) -> (-99.3, 8.3)
  line L9 (-99.3, 8.3) -> (-99.3, 1.6)
  line L10 (-99.3, 1.6) -> (-109.65, 1.6)
  line L11 (-109.65, 1.6) -> (-109.65, 34.9)
  line L12 (-109.65, 34.9) -> (-111.4, 34.9)
  line L13 (-111.4, 34.9) -> (-111.4, 0)
  line L14 (-111.4, 0) -> (0, 0)
  line L15 (0, 0) -> (0, 71.5)
  line L16 (0, 71.5) -> (-6, 71.5)
  line L17 (-6, 71.5) -> (-6, 93.5)
  line L18 (-6, 93.5) -> (-30.5, 93.5)
  line L19 (-30.5, 93.5) -> (-30.5, 58.65)
  line L20 (-30.5, 58.65) -> (-13.4, 58.65)
  line L21 (-13.4, 58.65) -> (-13.4, 62.65)
  line L22 (-13.4, 62.65) -> (-8.35, 62.65)
  line L23 (-8.35, 62.65) -> (-8.35, 58.65)
  line L24 (-8.35, 58.65) -> (-1.95, 58.65)
  line L25 (-1.95, 58.65) -> (-1.95, 47.65)
  line L26 (-1.95, 47.65) -> (-8.35, 47.65)
  line L27 (-8.35, 47.65) -> (-8.35, 43.65)
  line L28 (-8.35, 43.65) -> (-13.4, 43.65)
  line L29 (-13.4, 43.65) -> (-13.4, 47.65)
  line L30 (-13.4, 47.65) -> (-30.5, 47.65)
  line L31 (-30.5, 47.65) -> (-30.5, 34.2)
  circle A0 centre (-8.25, 35.175) radius 1.5
  line L32 (-13.4, 7.7) -> (-13.4, 11.7)
  line L33 (-13.4, 11.7) -> (-21.95, 11.7)
  line L34 (-21.95, 11.7) -> (-21.95, 22.7)
  line L35 (-21.95, 22.7) -> (-13.4, 22.7)
  line L36 (-13.4, 22.7) -> (-13.4, 26.7)
  line L37 (-13.4, 26.7) -> (-8.35, 26.7)
  line L38 (-8.35, 26.7) -> (-8.35, 22.7)
  line L39 (-8.35, 22.7) -> (-1.95, 22.7)
  line L40 (-1.95, 22.7) -> (-1.95, 11.7)
  line L41 (-1.95, 11.7) -> (-8.35, 11.7)
  line L42 (-8.35, 11.7) -> (-8.35, 7.7)
  line L43 (-8.35, 7.7) -> (-13.4, 7.7)
  circle A1 centre (-22.85, 35.175) radius 1.1
  dimension "d149" = 2.2
  dimension "d150" = 22.85
  constraint horizontal A0.centre A1.centre
  measures "d149" diameter of A1
  measures "d150" distance of L15 A1.centre
extrude "Extrude27" cut sketch "Sketch12" against normal blind 31 contours A1
sketch "Sketch14" plane through (0, 0, 19.1) normal (0, 0, -1) x (-1, 0, 0)
  line L0 (-98.4, 71.5) -> (-111.4, 71.5)
  line L1 (-111.4, 71.5) -> (-111.4, 34.9)
  line L2 (-111.4, 34.9) -> (-109.65, 34.9)
  line L3 (-109.65, 34.9) -> (-109.65, 1.6)
  line L4 (-109.65, 1.6) -> (-99.3, 1.6)
  line L5 (-99.3, 1.6) -> (-99.3, 8.3)
  line L6 (-99.3, 8.3) -> (-93.7, 8.3)
  line L7 (-93.7, 8.3) -> (-93.7, 26.1)
  line L8 (-93.7, 26.1) -> (-98.4, 26.1)
  line L9 (-98.4, 26.1) -> (-98.4, 71.5)
  circle A0 centre (-104.15, 26.7) radius 1.2
  circle A1 centre (-104.15, 7.7) radius 1.2
  line L10 (-111.4, 0) -> (-111.4, 34.9)
  line L11 (0, 0) -> (-111.4, 0)
  line L12 (-104.15, 26.7) -> (-104.15, 7.7) construction
  line L13 (-45.8, 8.3) -> (-45.8, 26.1) construction
  point P0 (-104.15, 17.2)
  point P1 (-45.8, 17.2)
  dimension "d156" = 19
  dimension "d157" = 7.25
  dimension "d159" = 2.4
  constraint vertical A0.centre A1.centre
  constraint equal A0 A1
  constraint coincident A0.centre L12.start
  constraint coincident A1.centre L12.end
  constraint midpoint L12 P0
  constraint midpoint L13 P1
  constraint horizontal P0 P1
  measures "d156" distance of A0.centre A1.centre
  measures "d157" distance of A0.centre L10
  measures "d159" diameter of A0
extrude "Extrude29" cut sketch "Sketch14" against normal blind 7.25 contours A0 | A1
sketch "Sketch15" plane through (0, 93.5, 0) normal (0, 1, 0) x (-1, 0, 0)
  line L0 (-98.4, 4.5) -> (-30.5, 4.5)
  line L1 (-30.5, 4.5) -> (-30.5, 0)
  line L2 (-30.5, 0) -> (-6, 0)
  line L3 (-6, 0) -> (-6, 42.8)
  line L4 (-6, 42.8) -> (-30.75, 42.8)
  line L5 (-30.75, 42.8) -> (-30.75, 33.3)
  line L6 (-30.75, 33.3) -> (-98.4, 33.3)
  line L7 (-98.4, 33.3) -> (-98.4, 4.5)
  circle A0 centre (-17.75, 0) radius 1.25
  circle A1 centre (-22.7, 25.7) radius 1.3
  circle A2 centre (-46.1, 25.7) radius 1.3
  circle A3 centre (-78, 12.2) radius 1.3
  circle A4 centre (-63.05, 10.55) radius 2
  line L8 (-65.05, 10.55) -> (-65.05, 0)
  line L9 (-61.05, 10.55) -> (-61.05, 0)
  circle A5 centre (-17.75, 0) radius 2.85
  line L10 (-30.5, 0) -> (-98.4, 0)
  circle A6 centre (-63.05, 10.55) radius 1.75
  line L11 (-98.4, 12.55) -> (-92.05, 12.55)
  line L12 (-92.05, 12.55) -> (-92.05, 0)
  circle A7 centre (-94.05, 10.55) radius 1.75
  line L13 (-94.05, 10.55) -> (-94.05, 12.55) construction
  line L14 (-94.05, 10.55) -> (-92.05, 10.55) construction
  line L15 (-92.05, 0) -> (-98.4, 0)
  line L16 (-98.4, 0) -> (-98.4, 12.55)
  point P0 (-63.05, 12.55)
  dimension "d162" = 4
  dimension "d165" = 20.4
  dimension "d166" = 7.7
  dimension "d167" = 2.6
  dimension "d168" = 2.6
  dimension "d169" = 7.6
  dimension "d170" = 40.1
  dimension "d171" = 16.7
  dimension "d172" = 2.5
  dimension "d173" = 11.75
  dimension "d174" = 5.7
  constraint coincident L2 A0.centre
  constraint coincident A4 L8.start
  constraint tangent A4 L8
  constraint perpendicular L0 L8
  constraint coincident A4 L9.start
  constraint tangent A4 L9
  constraint perpendicular L0 L9
  constraint horizontal A1.centre A2.centre
  constraint equal A1 A2
  constraint concentric A0 A5
  constraint coincident L8.end L10
  constraint coincident L9.end L10
  constraint concentric A4 A6
  constraint coincident L7 L11.start
  constraint perpendicular L7 L11
  constraint perpendicular L0 L12
  constraint coincident A4 P0
  constraint vertical A4.centre P0
  constraint horizontal L11.end P0
  constraint coincident A7.centre L13.start
  constraint coincident L11 L13.end
  constraint perpendicular L11 L13
  constraint coincident L12 L14.end
  constraint perpendicular L12 L14
  constraint equal L13 L14
  constraint coincident L10 L12.end
  constraint coincident L10.end L15.end
  measures "d162" diameter of A4
  measures "d165" distance of L7 A3.centre
  measures "d166" distance of L0 A3.centre
  measures "d167" diameter of A3
  measures "d168" diameter of A2
  measures "d169" distance of L6 A2.centre
  measures "d170" distance of L3 A2.centre
  measures "d171" distance of L3 A1.centre
  measures "d172" diameter of A0
  measures "d173" distance of L3 A0.centre
  measures "d174" diameter of A5
extrude "Extrude31" cut sketch "Sketch15" against normal blind 10 contours A1 | A2 | A3
extrude "Extrude32" cut sketch "Sketch15" against normal up to surface (67.4 mm away) contours L0 L7 L11 L12 L16 | L0 L10 L12 L15 L16 | L0 A4 L8 L9 | L0 L8 L9 L10 | A4 | A6 | A7
sketch "Sketch16" plane through (0, 0, 0) normal (-1, 0, 0) x (0, 0, 1)
  line L0 (0, 71.5) -> (0, 0)
  line L1 (0, 0) -> (42.8, 0)
  line L2 (42.8, 0) -> (42.8, 71.5)
  line L3 (42.8, 71.5) -> (0, 71.5)
  circle A0 centre (19.975, 42.825) radius 1.325
  circle A1 centre (19.975, 42.825) radius 3
  line L4 (42.8, 44.575) -> (22.4117, 44.575)
  line L5 (22.4117, 41.075) -> (42.8, 41.075)
  line L6 (42.8, 44.575) -> (42.8, 41.075)
  dimension "d182" = 2.65
  dimension "d183" = 6
  dimension "d184" = 3.5
  dimension "d185" = 22.825
  dimension "d186" = 28.675
  constraint concentric A0 A1
  constraint coincident L2 L4.start
  constraint coincident A1 L4.end
  constraint perpendicular L2 L4
  constraint coincident A1 L5.start
  constraint coincident L2 L5.end
  constraint perpendicular L2 L5
  constraint vertical L4.end L5.start
  measures "d182" diameter of A0
  measures "d183" diameter of A1
  measures "d184" distance of L4 L5
  measures "d185" distance of L2 A0.centre
  measures "d186" distance of L3 A0.centre
extrude "Extrude33" cut sketch "Sketch16" against normal blind 2.1 contours L2 A1 L4 L5 L6
extrude "Extrude34" add sketch "Sketch16" along normal blind 1 contours A1
extrude "Extrude35" cut sketch "Sketch16" against normal up to surface (2.95 mm away) from surface at 1 contours A0
fillet "Fillet1" radius 1.5 1 edges at (92.05, 59.8, 12.55)
chamfer "Chamfer5" distance 9.2 angle 45 1 edges at (0, 35.75, 0)